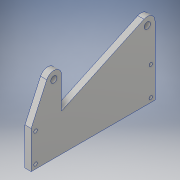
# Autodesk Inventor part: Intake Mount
Saved by Autodesk Inventor 2019.4 (Build 234330000, 330)
## iProperties
Created: 2020-01-06
Part Number: Intake Mount
Material: Aluminum 6061
Document SubType Name: Modeling
Designer: admin
Density: 2.7 g/cm^3
Appearance: Aluminum - Flat
Author: admin
Autodesk Inventor part; units mm, degrees
ref_plane "YZ Plane" through (0, 0, 0) normal (1, 0, 0) x (0, 1, 0)
ref_plane "XZ Plane" through (0, 0, 0) normal (0, 1, 0) x (-1, 0, 0)
ref_plane "XY Plane" through (0, 0, 0) normal (0, 0, 1) x (1, 0, 0)
sketch "Sketch1" plane through (0, 0, 0) normal (1, 0, 0) x (0, 1, 0)
  line L0 (0, 0) -> (0, -198.8852)
  circle A0 centre (110, -186.3852) radius 5
  arc A1 (121.3395, -181.1254) -> (110, -198.8852) centre (110, -186.3852) ccw construction
  circle A2 centre (110, -36.3852) radius 5
  arc A3 (110, -48.8852) -> (115.1601, -25) centre (110, -36.3852) ccw
  line L1 (0, 0) -> (60, 0)
  line L2 (60, 0) -> (115.1601, -25)
  line L3 (110, -48.8852) -> (60, -48.8852)
  line L4 (60, -48.8852) -> (121.3395, -181.1254)
  line L5 (110, -198.8852) -> (0, -198.8852)
  line L6 (110, -36.3852) -> (110, -186.3852) construction
  arc A4 (115.1601, -25) -> (110, -48.8852) centre (110, -36.3852) ccw construction
  arc A5 (110, -198.8852) -> (121.3395, -181.1254) centre (110, -186.3852) ccw
  line L7 (60, 0) -> (60, -48.8852) construction
  circle A6 centre (7, -7) radius 2.75
  circle A7 centre (53, -7) radius 2.75
  circle A8 centre (53, -191.8852) radius 2.75
  circle A9 centre (7, -191.8852) radius 2.75
  dimension "d0" = 10
  dimension "d1" = 25
  dimension "d2" = 25
  dimension "d3" = 10
  dimension "d4" = 60
  dimension "d5" = 150
  dimension "d6" = 50
  dimension "d7" = 25
  dimension "d8" = 5.5
  dimension "d9" = 5.5
  dimension "d10" = 5.5
  dimension "d11" = 5.5
  dimension "d12" = 7
  dimension "d13" = 7
  dimension "d14" = 7
  dimension "d15" = 7
  dimension "d16" = 7
  dimension "d17" = 7
  dimension "d18" = 7
  dimension "d19" = 7
  constraints: 16 end point, 10 centre point, 8 point on circle, 4 tangent, 3 vertical, 2 coincident, 2 horizontal, 1 perpendicular, 1 point on line
  measures "d0" diameter of A2
  measures "d1" diameter of A3
  measures "d2" diameter of A1
  measures "d3" diameter of A0
  measures "d4" distance of L0.start L1.end
  measures "d5" distance of L6.start L6.end
  measures "d6" distance from line of L1.end L6
  measures "d7" vertical distance of L1.end L2.end
  measures "d8" diameter of A6
  measures "d9" diameter of A7
  measures "d10" diameter of A8
  measures "d11" diameter of A9
  measures "d12" distance from line of L0 A6.centre
  measures "d13" distance from line of L1 A6.centre
  measures "d14" distance from line of L1 A7.centre
  measures "d15" distance from line of L7 A7.centre
  measures "d16" distance from line of L5 A8.centre
  measures "d17" distance from line of L5 A9.centre
  measures "d18" distance from line of L0 A9.centre
  measures "d19" distance from line of L7 A8.centre
extrude "Extrusion1" add sketch "Sketch1" along normal blind 10
body "Solid1"
